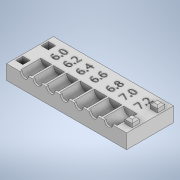
# Autodesk Inventor part: Measurement Test
Saved by Autodesk Inventor 2021 (Build 250183000, 183)
## iProperties
Created: 2021-06-07
Part Number: Measurement Test
Material: Generic
Document SubType Name: Modeling
Designer: Anton
Density: 1 g/cm^3
Appearance: Default
Author: Anton
Autodesk Inventor part; units mm, degrees
ref_plane "YZ Plane" through (0, 0, 0) normal (1, 0, 0) x (0, 1, 0)
ref_plane "XZ Plane" through (0, 0, 0) normal (0, 1, 0) x (-1, 0, 0)
ref_plane "XY Plane" through (0, 0, 0) normal (0, 0, 1) x (1, 0, 0)
sketch "Sketch1" plane through (0, 0, 0) normal (0, 1, 0) x (-1, 0, 0)
  line L0 (0, 0) -> (56, 0)
  line L1 (56, 0) -> (56, -15)
  line L2 (56, -15) -> (0, -15)
  line L3 (0, -15) -> (0, 0)
  dimension "d0" = 15
  dimension "d1" = 56
  constraints: 8 end point, 2 parallel, 1 horizontal, 1 perpendicular
  measures "d0" distance between parallel lines of L2 L0
  measures "d1" distance between parallel lines of L3 L1
extrude "Extrusion1" add sketch "Sketch1" along normal blind 8
sketch "Sketch2" plane through (-56, 0, 0) normal (0, 0, 1) x (1, 0, 0)
  line L0 (56, 8) -> (0, 8) projected
  circle A0 centre (4.85, 8) radius 3
  circle A1 centre (11.95, 8) radius 3.1
  circle A2 centre (19.25, 8) radius 3.2
  circle A3 centre (26.85, 8) radius 3.4
  circle A4 centre (34.75, 8) radius 3.5
  circle A5 centre (42.85, 8) radius 3.6
  line L1 (0, 0) -> (0, 8) projected
  line L2 (56, 0) -> (56, 8) projected
  circle A6 centre (51.15, 8) radius 3.7
  point P0 (47.45, 8)
  point P1 (54.85, 8)
  point P2 (39.25, 8)
  point P3 (46.45, 8)
  point P4 (31.25, 8)
  point P5 (38.25, 8)
  point P6 (23.45, 8)
  point P7 (30.25, 8)
  point P8 (16.05, 8)
  point P9 (22.45, 8)
  point P10 (8.85, 8)
  point P11 (15.05, 8)
  point P12 (1.85, 8)
  point P13 (7.85, 8)
  dimension "d4" = 6
  dimension "d5" = 6.2
  dimension "d6" = 6.4
  dimension "d7" = 6.8
  dimension "d8" = 7
  dimension "d9" = 7.2
  dimension "d10" = 4.85
  dimension "d12" = 1
  dimension "d13" = 1
  dimension "d14" = 1
  dimension "d15" = 1
  dimension "d17" = 1
  dimension "d18" = 7.4
  dimension "d19" = 1
  constraints: 7 centre point, 8 other
  measures "d4" diameter of A0
  measures "d5" diameter of A1
  measures "d6" diameter of A2
  measures "d7" diameter of A3
  measures "d8" diameter of A4
  measures "d9" diameter of A5
  measures "d10" distance from line of L1 A0.centre
  measures "d18" diameter of A6
extrude "Extrusion2" cut sketch "Sketch2" against normal blind 11 contours A6 L0 | A5 L0 | A4 L0 | A3 L0 | A2 L0 | A1 L0 | A0 L0 picked at (52.0195, 5.594) picked at (43.6691, 6.4548) picked at (34.8906, 6.8418) picked at (25.8719, 6.7218) picked at (18.6441, 7.1222) picked at (12.0746, 6.9742) picked at (5.7645, 7.296)
sketch "Sketch3" plane through (0, 8, 0) normal (0, 1, 0) x (1, 0, 0)
  line L0 (0, 0) -> (0, 15) projected
  line L1 (0, 15) -> (-55.9832, 15)
  line L2 (-55.9832, 15) -> (-55.9832, 24.7648)
  line L3 (-55.9832, 24.7648) -> (0, 24.7648)
  line L4 (0, 24.7648) -> (0, 15)
  constraints: 8 end point, 2 parallel, 1 horizontal, 1 perpendicular
extrude "Extrusion3" add sketch "Sketch3" against normal blind 8
sketch "Sketch5" plane through (0, 8, 0) normal (0, 1, 0) x (1, 0, 0)
  line L0 (-56, 15) -> (-56, 0) projected
  line L1 (-52.9832, 14) -> (-52.9832, 59.4153) construction
  line L2 (-52.9832, 59.4153) -> (-39.3814, 59.4153) construction
  line L3 (-39.3814, 59.4153) -> (-39.3814, 14) construction
  line L4 (-39.3814, 14) -> (-52.9832, 14) construction
  line L5 (-45.9832, 14) -> (-45.9832, 59.5193) construction
  line L6 (-45.9832, 59.5193) -> (-29.8115, 59.5193) construction
  line L7 (-29.8115, 59.5193) -> (-29.8115, 14) construction
  line L8 (-29.8115, 14) -> (-45.9832, 14) construction
  line L9 (-38.9832, 14) -> (-38.9832, 59.5309) construction
  line L10 (-38.9832, 59.5309) -> (-25.3814, 59.5309) construction
  line L11 (-25.3814, 59.5309) -> (-25.3814, 14) construction
  line L12 (-25.3814, 14) -> (-38.9832, 14) construction
  line L13 (-31.4832, 14) -> (-31.4832, 59.7081) construction
  line L14 (-31.4832, 59.7081) -> (-17.4293, 59.7081) construction
  line L15 (-17.4293, 59.7081) -> (-17.4293, 14) construction
  line L16 (-17.4293, 14) -> (-31.4832, 14) construction
  line L17 (-22.5355, 14) -> (-22.5355, 61.7081) construction
  line L18 (-22.5355, 61.7081) -> (-24.1276, 61.7081) construction
  line L19 (-24.1276, 61.7081) -> (-24.1276, 14) construction
  line L20 (-24.1276, 14) -> (-22.5355, 14) construction
  line L21 (-6.6524, 14) -> (-6.6524, 61.7081) construction
  line L22 (-6.6524, 61.7081) -> (6.9493, 61.7081) construction
  line L23 (6.9493, 61.7081) -> (6.9493, 14) construction
  line L24 (6.9493, 14) -> (-6.6524, 14) construction
  line L25 (-14.972, 14) -> (-14.972, 61.7081) construction
  line L26 (-14.972, 61.7081) -> (-1.3703, 61.7081) construction
  line L27 (-1.3703, 61.7081) -> (-1.3703, 14) construction
  line L28 (-1.3703, 14) -> (-14.972, 14) construction
  line L29 (-55.9832, 24.7648) -> (-55.9832, 15) projected
  line L30 (-48.15, 0) -> (-54.15, 0) projected
  line L31 (-40.95, 0) -> (-47.15, 0) projected
  line L32 (-33.55, 0) -> (-39.95, 0) projected
  line L33 (-25.75, 0) -> (-32.55, 0) projected
  line L34 (-9.55, 0) -> (-16.75, 0) projected
  line L35 (-1.15, 0) -> (-8.55, 0) projected
  line L36 (-17.75, 0) -> (-24.75, 0) projected
  line L37 (-5.9685, 16.8039) -> (-2.5681, 15.0729)
  line L38 (-2.5681, 15.0729) -> (-2.5681, 14.5024)
  line L39 (-2.5681, 14.5024) -> (-6.0981, 16.3306)
  line L40 (-6.0981, 16.3306) -> (-6.0981, 14.2658)
  line L41 (-6.0981, 14.2658) -> (-6.5681, 14.2658)
  line L42 (-6.5681, 14.2658) -> (-6.5681, 16.8039)
  line L43 (-6.5681, 16.8039) -> (-5.9685, 16.8039)
  line L44 (-2.5681, 18.1524) -> (-2.5681, 17.5105)
  line L45 (-2.5681, 17.5105) -> (-3.3331, 17.5105)
  line L46 (-3.3331, 17.5105) -> (-3.3331, 18.1524)
  line L47 (-3.3331, 18.1524) -> (-2.5681, 18.1524)
  line L48 (-2.5681, 21.4263) -> (-2.5681, 18.9595)
  line L49 (-2.5681, 18.9595) -> (-3.1354, 18.9595)
  spline S0 degree 2 poles (-3.1354, 18.9595) (-3.385, 19.2253) (-3.8485, 19.6985) (-4.0981, 19.9254) knots 0 0 0 1 2 2 2
  spline S1 degree 2 poles (-4.0981, 19.9254) (-4.6005, 20.3825) (-5.2035, 20.7164) (-5.5244, 20.7164) knots 0 0 0 1 2 2 2
  spline S2 degree 2 poles (-5.5244, 20.7164) (-5.6929, 20.7164) (-5.9458, 20.6126) (-6.0268, 20.5186) knots 0 0 0 1 2 2 2
  spline S3 degree 2 poles (-6.0268, 20.5186) (-6.1078, 20.4246) (-6.1889, 20.1783) (-6.1889, 20.0292) knots 0 0 0 1 2 2 2
  spline S4 degree 2 poles (-6.1889, 20.0292) (-6.1889, 19.8865) (-6.1176, 19.5948) (-6.0625, 19.4619) knots 0 0 0 1 2 2 2
  spline S5 degree 2 poles (-6.0625, 19.4619) (-6.0171, 19.3485) (-5.8874, 19.1378) (-5.842, 19.0729) knots 0 0 0 1 2 2 2
  line L50 (-5.842, 19.0729) -> (-5.842, 19.0438)
  line L51 (-5.842, 19.0438) -> (-6.4125, 19.0438)
  spline S6 degree 2 poles (-6.4125, 19.0438) (-6.4936, 19.2091) (-6.6524, 19.8023) (-6.6524, 20.0681) knots 0 0 0 1 2 2 2
  spline S7 degree 2 poles (-6.6524, 20.0681) (-6.6524, 20.6288) (-6.0592, 21.2609) (-5.5535, 21.2609) knots 0 0 0 1 2 2 2
  spline S8 degree 2 poles (-5.5535, 21.2609) (-5.3169, 21.2609) (-4.9214, 21.1507) (-4.7529, 21.0535) knots 0 0 0 1 2 2 2
  spline S9 degree 2 poles (-4.7529, 21.0535) (-4.5779, 20.9562) (-4.2343, 20.6742) (-4.0689, 20.5186) knots 0 0 0 1 2 2 2
  spline S10 degree 2 poles (-4.0689, 20.5186) (-3.7934, 20.2658) (-3.2035, 19.6467) (-3.0317, 19.4619) knots 0 0 0 1 2 2 2
  line L52 (-3.0317, 19.4619) -> (-3.0317, 21.4263)
  line L53 (-3.0317, 21.4263) -> (-2.5681, 21.4263)
  line L54 (-14.2913, 16.8039) -> (-10.891, 15.0729)
  line L55 (-10.891, 15.0729) -> (-10.891, 14.5024)
  line L56 (-10.891, 14.5024) -> (-14.421, 16.3306)
  line L57 (-14.421, 16.3306) -> (-14.421, 14.2658)
  line L58 (-14.421, 14.2658) -> (-14.891, 14.2658)
  line L59 (-14.891, 14.2658) -> (-14.891, 16.8039)
  line L60 (-14.891, 16.8039) -> (-14.2913, 16.8039)
  line L61 (-10.891, 18.1524) -> (-10.891, 17.5105)
  line L62 (-10.891, 17.5105) -> (-11.656, 17.5105)
  line L63 (-11.656, 17.5105) -> (-11.656, 18.1524)
  line L64 (-11.656, 18.1524) -> (-10.891, 18.1524)
  spline S11 degree 2 poles (-12.891, 21.4489) (-11.8148, 21.4489) (-10.8067, 20.8233) (-10.8067, 20.1718) knots 0 0 0 1 2 2 2
  spline S12 degree 2 poles (-10.8067, 20.1718) (-10.8067, 19.5105) (-11.8342, 18.8914) (-12.8877, 18.8914) knots 0 0 0 1 2 2 2
  spline S13 degree 2 poles (-12.8877, 18.8914) (-13.9704, 18.8914) (-14.972, 19.517) (-14.972, 20.1718) knots 0 0 0 1 2 2 2
  spline S14 degree 2 poles (-14.972, 20.1718) (-14.972, 20.8298) (-13.9347, 21.4489) (-12.891, 21.4489) knots 0 0 0 1 2 2 2
  spline S15 degree 2 poles (-11.6722, 20.7618) (-11.8699, 20.8395) (-12.4793, 20.9044) (-12.891, 20.9044) knots 0 0 0 1 2 2 2
  spline S16 degree 2 poles (-12.891, 20.9044) (-13.3026, 20.9044) (-13.9088, 20.8395) (-14.113, 20.7585) knots 0 0 0 1 2 2 2
  spline S17 degree 2 poles (-14.113, 20.7585) (-14.3172, 20.6775) (-14.5279, 20.3955) (-14.5279, 20.1718) knots 0 0 0 1 2 2 2
  spline S18 degree 2 poles (-14.5279, 20.1718) (-14.5279, 19.9481) (-14.3172, 19.6596) (-14.1065, 19.5754) knots 0 0 0 1 2 2 2
  spline S19 degree 2 poles (-14.1065, 19.5754) (-13.9023, 19.4943) (-13.2799, 19.436) (-12.8877, 19.436) knots 0 0 0 1 2 2 2
  spline S20 degree 2 poles (-12.8877, 19.436) (-12.4663, 19.436) (-11.9023, 19.4878) (-11.6819, 19.5721) knots 0 0 0 1 2 2 2
  spline S21 degree 2 poles (-11.6819, 19.5721) (-11.4744, 19.6499) (-11.2508, 19.9384) (-11.2508, 20.1718) knots 0 0 0 1 2 2 2
  spline S22 degree 2 poles (-11.2508, 20.1718) (-11.2508, 20.3922) (-11.4615, 20.6807) (-11.6722, 20.7618) knots 0 0 0 1 2 2 2
  spline S23 degree 2 poles (-19.7414, 16.8201) (-19.4334, 16.8201) (-18.9115, 16.6159) (-18.7365, 16.4441) knots 0 0 0 1 2 2 2
  spline S24 degree 2 poles (-18.7365, 16.4441) (-18.5517, 16.2658) (-18.3605, 15.8185) (-18.3605, 15.5494) knots 0 0 0 1 2 2 2
  spline S25 degree 2 poles (-18.3605, 15.5494) (-18.3605, 15.2804) (-18.542, 14.8363) (-18.7235, 14.6677) knots 0 0 0 1 2 2 2
  spline S26 degree 2 poles (-18.7235, 14.6677) (-18.9407, 14.4603) (-19.67, 14.2269) (-20.2017, 14.2269) knots 0 0 0 1 2 2 2
  spline S27 degree 2 poles (-20.2017, 14.2269) (-20.7235, 14.2269) (-21.5631, 14.4408) (-21.8743, 14.6645) knots 0 0 0 1 2 2 2
  spline S28 degree 2 poles (-21.8743, 14.6645) (-22.179, 14.8817) (-22.5193, 15.5689) (-22.5193, 16.0194) knots 0 0 0 1 2 2 2
  spline S29 degree 2 poles (-22.5193, 16.0194) (-22.5193, 16.1524) (-22.4934, 16.3857) (-22.4642, 16.4733) knots 0 0 0 1 2 2 2
  line L65 (-22.4642, 16.4733) -> (-21.9488, 16.4733)
  line L66 (-21.9488, 16.4733) -> (-21.9488, 16.4506)
  spline S30 degree 2 poles (-21.9488, 16.4506) (-21.9877, 16.376) (-22.0558, 16.1037) (-22.0558, 15.9481) knots 0 0 0 1 2 2 2
  spline S31 degree 2 poles (-22.0558, 15.9481) (-22.0558, 15.4489) (-21.3816, 14.8363) (-20.7203, 14.778) knots 0 0 0 1 2 2 2
  spline S32 degree 2 poles (-20.7203, 14.778) (-20.8532, 14.9692) (-20.9991, 15.3712) (-20.9991, 15.611) knots 0 0 0 1 2 2 2
  spline S33 degree 2 poles (-20.9991, 15.611) (-20.9991, 15.8444) (-20.9051, 16.1945) (-20.7624, 16.3857) knots 0 0 0 1 2 2 2
  spline S34 degree 2 poles (-20.7624, 16.3857) (-20.5971, 16.6062) (-20.085, 16.8201) (-19.7414, 16.8201) knots 0 0 0 1 2 2 2
  spline S35 degree 2 poles (-19.7187, 16.2755) (-19.965, 16.2755) (-20.2989, 16.1459) (-20.4156, 16.0032) knots 0 0 0 1 2 2 2
  spline S36 degree 2 poles (-20.4156, 16.0032) (-20.4999, 15.8963) (-20.555, 15.6305) (-20.555, 15.4911) knots 0 0 0 1 2 2 2
  spline S37 degree 2 poles (-20.555, 15.4911) (-20.555, 15.3031) (-20.4415, 14.9498) (-20.3346, 14.778) knots 0 0 0 1 2 2 2
  spline S38 degree 2 poles (-20.3346, 14.778) (-20.2762, 14.7747) (-20.166, 14.7682) (-20.0817, 14.7682) knots 0 0 0 1 2 2 2
  spline S39 degree 2 poles (-20.0817, 14.7682) (-19.6668, 14.7682) (-19.1579, 14.9303) (-19.025, 15.0535) knots 0 0 0 1 2 2 2
  spline S40 degree 2 poles (-19.025, 15.0535) (-18.8986, 15.1669) (-18.7981, 15.4133) (-18.7981, 15.5527) knots 0 0 0 1 2 2 2
  spline S41 degree 2 poles (-18.7981, 15.5527) (-18.7981, 15.8768) (-19.2584, 16.2755) (-19.7187, 16.2755) knots 0 0 0 1 2 2 2
  line L67 (-18.4448, 18.1524) -> (-18.4448, 17.5105)
  line L68 (-18.4448, 17.5105) -> (-19.2098, 17.5105)
  line L69 (-19.2098, 17.5105) -> (-19.2098, 18.1524)
  line L70 (-19.2098, 18.1524) -> (-18.4448, 18.1524)
  spline S42 degree 2 poles (-18.354, 20.1686) (-18.354, 19.8703) (-18.5323, 19.3809) (-18.6976, 19.2091) knots 0 0 0 1 2 2 2
  spline S43 degree 2 poles (-18.6976, 19.2091) (-18.8597, 19.0405) (-19.3005, 18.8655) (-19.5501, 18.8655) knots 0 0 0 1 2 2 2
  spline S44 degree 2 poles (-19.5501, 18.8655) (-19.8743, 18.8655) (-20.4188, 19.2123) (-20.5809, 19.5429) knots 0 0 0 1 2 2 2
  line L71 (-20.5809, 19.5429) -> (-20.5971, 19.5429)
  spline S45 degree 2 poles (-20.5971, 19.5429) (-20.7689, 19.248) (-21.1773, 18.9627) (-21.482, 18.9627) knots 0 0 0 1 2 2 2
  spline S46 degree 2 poles (-21.482, 18.9627) (-21.9326, 18.9627) (-22.5355, 19.6434) (-22.5355, 20.1686) knots 0 0 0 1 2 2 2
  spline S47 degree 2 poles (-22.5355, 20.1686) (-22.5355, 20.7131) (-21.965, 21.3712) (-21.5177, 21.3712) knots 0 0 0 1 2 2 2
  spline S48 degree 2 poles (-21.5177, 21.3712) (-21.2487, 21.3712) (-20.7235, 21.0567) (-20.5744, 20.7618) knots 0 0 0 1 2 2 2
  line L72 (-20.5744, 20.7618) -> (-20.5582, 20.7618)
  spline S49 degree 2 poles (-20.5582, 20.7618) (-20.3961, 21.1118) (-19.9294, 21.4716) (-19.5598, 21.4716) knots 0 0 0 1 2 2 2
  spline S50 degree 2 poles (-19.5598, 21.4716) (-19.0477, 21.4716) (-18.354, 20.7261) (-18.354, 20.1686) knots 0 0 0 1 2 2 2
  spline S51 degree 2 poles (-19.508, 20.9206) (-19.7543, 20.9206) (-20.0461, 20.7261) (-20.1952, 20.4506) knots 0 0 0 1 2 2 2
  spline S52 degree 2 poles (-20.1952, 20.4506) (-20.247, 20.3598) (-20.367, 20.0551) (-20.4448, 19.8639) knots 0 0 0 1 2 2 2
  spline S53 degree 2 poles (-20.4448, 19.8639) (-20.2989, 19.6434) (-19.8645, 19.4068) (-19.589, 19.4068) knots 0 0 0 1 2 2 2
  spline S54 degree 2 poles (-19.589, 19.4068) (-19.226, 19.4068) (-18.7527, 19.8444) (-18.7527, 20.175) knots 0 0 0 1 2 2 2
  spline S55 degree 2 poles (-18.7527, 20.175) (-18.7527, 20.5122) (-19.1579, 20.9206) (-19.508, 20.9206) knots 0 0 0 1 2 2 2
  spline S56 degree 2 poles (-21.5112, 20.846) (-21.7803, 20.846) (-22.1401, 20.4862) (-22.1401, 20.1653) knots 0 0 0 1 2 2 2
  spline S57 degree 2 poles (-22.1401, 20.1653) (-22.1401, 19.8736) (-21.8192, 19.5008) (-21.5436, 19.5008) knots 0 0 0 1 2 2 2
  spline S58 degree 2 poles (-21.5436, 19.5008) (-21.3459, 19.5008) (-21.0704, 19.6921) (-20.9602, 19.8833) knots 0 0 0 1 2 2 2
  spline S59 degree 2 poles (-20.9602, 19.8833) (-20.9148, 19.9643) (-20.7559, 20.3079) (-20.7106, 20.4473) knots 0 0 0 1 2 2 2
  spline S60 degree 2 poles (-20.7106, 20.4473) (-20.8888, 20.6807) (-21.2681, 20.846) (-21.5112, 20.846) knots 0 0 0 1 2 2 2
  spline S61 degree 2 poles (-28.7052, 16.8201) (-28.3973, 16.8201) (-27.8754, 16.6159) (-27.7003, 16.4441) knots 0 0 0 1 2 2 2
  spline S62 degree 2 poles (-27.7003, 16.4441) (-27.5156, 16.2658) (-27.3243, 15.8185) (-27.3243, 15.5494) knots 0 0 0 1 2 2 2
  spline S63 degree 2 poles (-27.3243, 15.5494) (-27.3243, 15.2804) (-27.5058, 14.8363) (-27.6874, 14.6677) knots 0 0 0 1 2 2 2
  spline S64 degree 2 poles (-27.6874, 14.6677) (-27.9046, 14.4603) (-28.6339, 14.2269) (-29.1655, 14.2269) knots 0 0 0 1 2 2 2
  spline S65 degree 2 poles (-29.1655, 14.2269) (-29.6874, 14.2269) (-30.5269, 14.4408) (-30.8381, 14.6645) knots 0 0 0 1 2 2 2
  spline S66 degree 2 poles (-30.8381, 14.6645) (-31.1428, 14.8817) (-31.4832, 15.5689) (-31.4832, 16.0194) knots 0 0 0 1 2 2 2
  spline S67 degree 2 poles (-31.4832, 16.0194) (-31.4832, 16.1524) (-31.4572, 16.3857) (-31.4281, 16.4733) knots 0 0 0 1 2 2 2
  line L73 (-31.4281, 16.4733) -> (-30.9127, 16.4733)
  line L74 (-30.9127, 16.4733) -> (-30.9127, 16.4506)
  spline S68 degree 2 poles (-30.9127, 16.4506) (-30.9516, 16.376) (-31.0196, 16.1037) (-31.0196, 15.9481) knots 0 0 0 1 2 2 2
  spline S69 degree 2 poles (-31.0196, 15.9481) (-31.0196, 15.4489) (-30.3454, 14.8363) (-29.6841, 14.778) knots 0 0 0 1 2 2 2
  spline S70 degree 2 poles (-29.6841, 14.778) (-29.817, 14.9692) (-29.9629, 15.3712) (-29.9629, 15.611) knots 0 0 0 1 2 2 2
  spline S71 degree 2 poles (-29.9629, 15.611) (-29.9629, 15.8444) (-29.8689, 16.1945) (-29.7263, 16.3857) knots 0 0 0 1 2 2 2
  spline S72 degree 2 poles (-29.7263, 16.3857) (-29.561, 16.6062) (-29.0488, 16.8201) (-28.7052, 16.8201) knots 0 0 0 1 2 2 2
  spline S73 degree 2 poles (-28.6825, 16.2755) (-28.9289, 16.2755) (-29.2627, 16.1459) (-29.3794, 16.0032) knots 0 0 0 1 2 2 2
  spline S74 degree 2 poles (-29.3794, 16.0032) (-29.4637, 15.8963) (-29.5188, 15.6305) (-29.5188, 15.4911) knots 0 0 0 1 2 2 2
  spline S75 degree 2 poles (-29.5188, 15.4911) (-29.5188, 15.3031) (-29.4054, 14.9498) (-29.2984, 14.778) knots 0 0 0 1 2 2 2
  spline S76 degree 2 poles (-29.2984, 14.778) (-29.24, 14.7747) (-29.1298, 14.7682) (-29.0456, 14.7682) knots 0 0 0 1 2 2 2
  spline S77 degree 2 poles (-29.0456, 14.7682) (-28.6306, 14.7682) (-28.1217, 14.9303) (-27.9888, 15.0535) knots 0 0 0 1 2 2 2
  spline S78 degree 2 poles (-27.9888, 15.0535) (-27.8624, 15.1669) (-27.7619, 15.4133) (-27.7619, 15.5527) knots 0 0 0 1 2 2 2
  spline S79 degree 2 poles (-27.7619, 15.5527) (-27.7619, 15.8768) (-28.2222, 16.2755) (-28.6825, 16.2755) knots 0 0 0 1 2 2 2
  line L75 (-27.4086, 18.1524) -> (-27.4086, 17.5105)
  line L76 (-27.4086, 17.5105) -> (-28.1736, 17.5105)
  line L77 (-28.1736, 17.5105) -> (-28.1736, 18.1524)
  line L78 (-28.1736, 18.1524) -> (-27.4086, 18.1524)
  spline S80 degree 2 poles (-28.7052, 21.4878) (-28.3973, 21.4878) (-27.8754, 21.2836) (-27.7003, 21.1118) knots 0 0 0 1 2 2 2
  spline S81 degree 2 poles (-27.7003, 21.1118) (-27.5156, 20.9335) (-27.3243, 20.4862) (-27.3243, 20.2172) knots 0 0 0 1 2 2 2
  spline S82 degree 2 poles (-27.3243, 20.2172) (-27.3243, 19.9481) (-27.5058, 19.5041) (-27.6874, 19.3355) knots 0 0 0 1 2 2 2
  spline S83 degree 2 poles (-27.6874, 19.3355) (-27.9046, 19.128) (-28.6339, 18.8947) (-29.1655, 18.8947) knots 0 0 0 1 2 2 2
  spline S84 degree 2 poles (-29.1655, 18.8947) (-29.6874, 18.8947) (-30.5269, 19.1086) (-30.8381, 19.3323) knots 0 0 0 1 2 2 2
  spline S85 degree 2 poles (-30.8381, 19.3323) (-31.1428, 19.5494) (-31.4832, 20.2366) (-31.4832, 20.6872) knots 0 0 0 1 2 2 2
  spline S86 degree 2 poles (-31.4832, 20.6872) (-31.4832, 20.8201) (-31.4572, 21.0535) (-31.4281, 21.141) knots 0 0 0 1 2 2 2
  line L79 (-31.4281, 21.141) -> (-30.9127, 21.141)
  line L80 (-30.9127, 21.141) -> (-30.9127, 21.1183)
  spline S87 degree 2 poles (-30.9127, 21.1183) (-30.9516, 21.0438) (-31.0196, 20.7715) (-31.0196, 20.6159) knots 0 0 0 1 2 2 2
  spline S88 degree 2 poles (-31.0196, 20.6159) (-31.0196, 20.1167) (-30.3454, 19.5041) (-29.6841, 19.4457) knots 0 0 0 1 2 2 2
  spline S89 degree 2 poles (-29.6841, 19.4457) (-29.817, 19.637) (-29.9629, 20.0389) (-29.9629, 20.2788) knots 0 0 0 1 2 2 2
  spline S90 degree 2 poles (-29.9629, 20.2788) (-29.9629, 20.5122) (-29.8689, 20.8622) (-29.7263, 21.0535) knots 0 0 0 1 2 2 2
  spline S91 degree 2 poles (-29.7263, 21.0535) (-29.561, 21.2739) (-29.0488, 21.4878) (-28.7052, 21.4878) knots 0 0 0 1 2 2 2
  spline S92 degree 2 poles (-28.6825, 20.9433) (-28.9289, 20.9433) (-29.2627, 20.8136) (-29.3794, 20.671) knots 0 0 0 1 2 2 2
  spline S93 degree 2 poles (-29.3794, 20.671) (-29.4637, 20.564) (-29.5188, 20.2982) (-29.5188, 20.1588) knots 0 0 0 1 2 2 2
  spline S94 degree 2 poles (-29.5188, 20.1588) (-29.5188, 19.9708) (-29.4054, 19.6175) (-29.2984, 19.4457) knots 0 0 0 1 2 2 2
  spline S95 degree 2 poles (-29.2984, 19.4457) (-29.24, 19.4425) (-29.1298, 19.436) (-29.0456, 19.436) knots 0 0 0 1 2 2 2
  spline S96 degree 2 poles (-29.0456, 19.436) (-28.6306, 19.436) (-28.1217, 19.5981) (-27.9888, 19.7212) knots 0 0 0 1 2 2 2
  spline S97 degree 2 poles (-27.9888, 19.7212) (-27.8624, 19.8347) (-27.7619, 20.081) (-27.7619, 20.2204) knots 0 0 0 1 2 2 2
  spline S98 degree 2 poles (-27.7619, 20.2204) (-27.7619, 20.5446) (-28.2222, 20.9433) (-28.6825, 20.9433) knots 0 0 0 1 2 2 2
  spline S99 degree 2 poles (-36.2052, 16.8201) (-35.8973, 16.8201) (-35.3754, 16.6159) (-35.2003, 16.4441) knots 0 0 0 1 2 2 2
  spline S100 degree 2 poles (-35.2003, 16.4441) (-35.0156, 16.2658) (-34.8243, 15.8185) (-34.8243, 15.5494) knots 0 0 0 1 2 2 2
  spline S101 degree 2 poles (-34.8243, 15.5494) (-34.8243, 15.2804) (-35.0058, 14.8363) (-35.1874, 14.6677) knots 0 0 0 1 2 2 2
  spline S102 degree 2 poles (-35.1874, 14.6677) (-35.4046, 14.4603) (-36.1339, 14.2269) (-36.6655, 14.2269) knots 0 0 0 1 2 2 2
  spline S103 degree 2 poles (-36.6655, 14.2269) (-37.1874, 14.2269) (-38.0269, 14.4408) (-38.3381, 14.6645) knots 0 0 0 1 2 2 2
  spline S104 degree 2 poles (-38.3381, 14.6645) (-38.6428, 14.8817) (-38.9832, 15.5689) (-38.9832, 16.0194) knots 0 0 0 1 2 2 2
  spline S105 degree 2 poles (-38.9832, 16.0194) (-38.9832, 16.1524) (-38.9572, 16.3857) (-38.9281, 16.4733) knots 0 0 0 1 2 2 2
  line L81 (-38.9281, 16.4733) -> (-38.4127, 16.4733)
  line L82 (-38.4127, 16.4733) -> (-38.4127, 16.4506)
  spline S106 degree 2 poles (-38.4127, 16.4506) (-38.4516, 16.376) (-38.5196, 16.1037) (-38.5196, 15.9481) knots 0 0 0 1 2 2 2
  spline S107 degree 2 poles (-38.5196, 15.9481) (-38.5196, 15.4489) (-37.8454, 14.8363) (-37.1841, 14.778) knots 0 0 0 1 2 2 2
  spline S108 degree 2 poles (-37.1841, 14.778) (-37.317, 14.9692) (-37.4629, 15.3712) (-37.4629, 15.611) knots 0 0 0 1 2 2 2
  spline S109 degree 2 poles (-37.4629, 15.611) (-37.4629, 15.8444) (-37.3689, 16.1945) (-37.2263, 16.3857) knots 0 0 0 1 2 2 2
  spline S110 degree 2 poles (-37.2263, 16.3857) (-37.061, 16.6062) (-36.5488, 16.8201) (-36.2052, 16.8201) knots 0 0 0 1 2 2 2
  spline S111 degree 2 poles (-36.1825, 16.2755) (-36.4289, 16.2755) (-36.7627, 16.1459) (-36.8794, 16.0032) knots 0 0 0 1 2 2 2
  spline S112 degree 2 poles (-36.8794, 16.0032) (-36.9637, 15.8963) (-37.0188, 15.6305) (-37.0188, 15.4911) knots 0 0 0 1 2 2 2
  spline S113 degree 2 poles (-37.0188, 15.4911) (-37.0188, 15.3031) (-36.9054, 14.9498) (-36.7984, 14.778) knots 0 0 0 1 2 2 2
  spline S114 degree 2 poles (-36.7984, 14.778) (-36.74, 14.7747) (-36.6298, 14.7682) (-36.5456, 14.7682) knots 0 0 0 1 2 2 2
  spline S115 degree 2 poles (-36.5456, 14.7682) (-36.1306, 14.7682) (-35.6217, 14.9303) (-35.4888, 15.0535) knots 0 0 0 1 2 2 2
  spline S116 degree 2 poles (-35.4888, 15.0535) (-35.3624, 15.1669) (-35.2619, 15.4133) (-35.2619, 15.5527) knots 0 0 0 1 2 2 2
  spline S117 degree 2 poles (-35.2619, 15.5527) (-35.2619, 15.8768) (-35.7222, 16.2755) (-36.1825, 16.2755) knots 0 0 0 1 2 2 2
  line L83 (-34.9086, 18.1524) -> (-34.9086, 17.5105)
  line L84 (-34.9086, 17.5105) -> (-35.6736, 17.5105)
  line L85 (-35.6736, 17.5105) -> (-35.6736, 18.1524)
  line L86 (-35.6736, 18.1524) -> (-34.9086, 18.1524)
  line L87 (-36.283, 21.5332) -> (-36.283, 21.0567)
  line L88 (-36.283, 21.0567) -> (-34.9086, 21.0567)
  line L89 (-34.9086, 21.0567) -> (-34.9086, 20.5413)
  line L90 (-34.9086, 20.5413) -> (-36.283, 20.5413)
  line L91 (-36.283, 20.5413) -> (-36.283, 18.7747)
  line L92 (-36.283, 18.7747) -> (-36.847, 18.7747)
  line L93 (-36.847, 18.7747) -> (-38.9086, 20.564)
  line L94 (-38.9086, 20.564) -> (-38.9086, 21.0567)
  line L95 (-38.9086, 21.0567) -> (-36.7141, 21.0567)
  line L96 (-36.7141, 21.0567) -> (-36.7141, 21.5332)
  line L97 (-36.7141, 21.5332) -> (-36.283, 21.5332)
  line L98 (-36.7141, 20.5413) -> (-38.2765, 20.5413)
  line L99 (-38.2765, 20.5413) -> (-36.7141, 19.1961)
  line L100 (-36.7141, 19.1961) -> (-36.7141, 20.5413)
  spline S118 degree 2 poles (-43.1955, 16.8201) (-42.8875, 16.8201) (-42.3657, 16.6159) (-42.1906, 16.4441) knots 0 0 0 1 2 2 2
  spline S119 degree 2 poles (-42.1906, 16.4441) (-42.0058, 16.2658) (-41.8146, 15.8185) (-41.8146, 15.5494) knots 0 0 0 1 2 2 2
  spline S120 degree 2 poles (-41.8146, 15.5494) (-41.8146, 15.2804) (-41.9961, 14.8363) (-42.1776, 14.6677) knots 0 0 0 1 2 2 2
  spline S121 degree 2 poles (-42.1776, 14.6677) (-42.3948, 14.4603) (-43.1242, 14.2269) (-43.6558, 14.2269) knots 0 0 0 1 2 2 2
  spline S122 degree 2 poles (-43.6558, 14.2269) (-44.1776, 14.2269) (-45.0172, 14.4408) (-45.3284, 14.6645) knots 0 0 0 1 2 2 2
  spline S123 degree 2 poles (-45.3284, 14.6645) (-45.6331, 14.8817) (-45.9734, 15.5689) (-45.9734, 16.0194) knots 0 0 0 1 2 2 2
  spline S124 degree 2 poles (-45.9734, 16.0194) (-45.9734, 16.1524) (-45.9475, 16.3857) (-45.9183, 16.4733) knots 0 0 0 1 2 2 2
  line L101 (-45.9183, 16.4733) -> (-45.4029, 16.4733)
  line L102 (-45.4029, 16.4733) -> (-45.4029, 16.4506)
  spline S125 degree 2 poles (-45.4029, 16.4506) (-45.4418, 16.376) (-45.5099, 16.1037) (-45.5099, 15.9481) knots 0 0 0 1 2 2 2
  spline S126 degree 2 poles (-45.5099, 15.9481) (-45.5099, 15.4489) (-44.8357, 14.8363) (-44.1744, 14.778) knots 0 0 0 1 2 2 2
  spline S127 degree 2 poles (-44.1744, 14.778) (-44.3073, 14.9692) (-44.4532, 15.3712) (-44.4532, 15.611) knots 0 0 0 1 2 2 2
  spline S128 degree 2 poles (-44.4532, 15.611) (-44.4532, 15.8444) (-44.3592, 16.1945) (-44.2165, 16.3857) knots 0 0 0 1 2 2 2
  spline S129 degree 2 poles (-44.2165, 16.3857) (-44.0512, 16.6062) (-43.5391, 16.8201) (-43.1955, 16.8201) knots 0 0 0 1 2 2 2
  spline S130 degree 2 poles (-43.1728, 16.2755) (-43.4191, 16.2755) (-43.753, 16.1459) (-43.8697, 16.0032) knots 0 0 0 1 2 2 2
  spline S131 degree 2 poles (-43.8697, 16.0032) (-43.954, 15.8963) (-44.0091, 15.6305) (-44.0091, 15.4911) knots 0 0 0 1 2 2 2
  spline S132 degree 2 poles (-44.0091, 15.4911) (-44.0091, 15.3031) (-43.8956, 14.9498) (-43.7887, 14.778) knots 0 0 0 1 2 2 2
  spline S133 degree 2 poles (-43.7887, 14.778) (-43.7303, 14.7747) (-43.6201, 14.7682) (-43.5358, 14.7682) knots 0 0 0 1 2 2 2
  spline S134 degree 2 poles (-43.5358, 14.7682) (-43.1209, 14.7682) (-42.612, 14.9303) (-42.4791, 15.0535) knots 0 0 0 1 2 2 2
  spline S135 degree 2 poles (-42.4791, 15.0535) (-42.3527, 15.1669) (-42.2522, 15.4133) (-42.2522, 15.5527) knots 0 0 0 1 2 2 2
  spline S136 degree 2 poles (-42.2522, 15.5527) (-42.2522, 15.8768) (-42.7125, 16.2755) (-43.1728, 16.2755) knots 0 0 0 1 2 2 2
  line L103 (-41.8989, 18.1524) -> (-41.8989, 17.5105)
  line L104 (-41.8989, 17.5105) -> (-42.6639, 17.5105)
  line L105 (-42.6639, 17.5105) -> (-42.6639, 18.1524)
  line L106 (-42.6639, 18.1524) -> (-41.8989, 18.1524)
  line L107 (-41.8989, 21.4263) -> (-41.8989, 18.9595)
  line L108 (-41.8989, 18.9595) -> (-42.4661, 18.9595)
  spline S137 degree 2 poles (-42.4661, 18.9595) (-42.7157, 19.2253) (-43.1793, 19.6985) (-43.4289, 19.9254) knots 0 0 0 1 2 2 2
  spline S138 degree 2 poles (-43.4289, 19.9254) (-43.9313, 20.3825) (-44.5342, 20.7164) (-44.8551, 20.7164) knots 0 0 0 1 2 2 2
  spline S139 degree 2 poles (-44.8551, 20.7164) (-45.0237, 20.7164) (-45.2765, 20.6126) (-45.3576, 20.5186) knots 0 0 0 1 2 2 2
  spline S140 degree 2 poles (-45.3576, 20.5186) (-45.4386, 20.4246) (-45.5196, 20.1783) (-45.5196, 20.0292) knots 0 0 0 1 2 2 2
  spline S141 degree 2 poles (-45.5196, 20.0292) (-45.5196, 19.8865) (-45.4483, 19.5948) (-45.3932, 19.4619) knots 0 0 0 1 2 2 2
  spline S142 degree 2 poles (-45.3932, 19.4619) (-45.3478, 19.3485) (-45.2182, 19.1378) (-45.1728, 19.0729) knots 0 0 0 1 2 2 2
  line L109 (-45.1728, 19.0729) -> (-45.1728, 19.0438)
  line L110 (-45.1728, 19.0438) -> (-45.7433, 19.0438)
  spline S143 degree 2 poles (-45.7433, 19.0438) (-45.8243, 19.2091) (-45.9832, 19.8023) (-45.9832, 20.0681) knots 0 0 0 1 2 2 2
  spline S144 degree 2 poles (-45.9832, 20.0681) (-45.9832, 20.6288) (-45.39, 21.2609) (-44.8843, 21.2609) knots 0 0 0 1 2 2 2
  spline S145 degree 2 poles (-44.8843, 21.2609) (-44.6477, 21.2609) (-44.2522, 21.1507) (-44.0836, 21.0535) knots 0 0 0 1 2 2 2
  spline S146 degree 2 poles (-44.0836, 21.0535) (-43.9086, 20.9562) (-43.565, 20.6742) (-43.3997, 20.5186) knots 0 0 0 1 2 2 2
  spline S147 degree 2 poles (-43.3997, 20.5186) (-43.1242, 20.2658) (-42.5342, 19.6467) (-42.3624, 19.4619) knots 0 0 0 1 2 2 2
  line L111 (-42.3624, 19.4619) -> (-42.3624, 21.4263)
  line L112 (-42.3624, 21.4263) -> (-41.8989, 21.4263)
  spline S148 degree 2 poles (-50.1987, 16.8201) (-49.8908, 16.8201) (-49.3689, 16.6159) (-49.1939, 16.4441) knots 0 0 0 1 2 2 2
  spline S149 degree 2 poles (-49.1939, 16.4441) (-49.0091, 16.2658) (-48.8178, 15.8185) (-48.8178, 15.5494) knots 0 0 0 1 2 2 2
  spline S150 degree 2 poles (-48.8178, 15.5494) (-48.8178, 15.2804) (-48.9994, 14.8363) (-49.1809, 14.6677) knots 0 0 0 1 2 2 2
  spline S151 degree 2 poles (-49.1809, 14.6677) (-49.3981, 14.4603) (-50.1274, 14.2269) (-50.659, 14.2269) knots 0 0 0 1 2 2 2
  spline S152 degree 2 poles (-50.659, 14.2269) (-51.1809, 14.2269) (-52.0204, 14.4408) (-52.3316, 14.6645) knots 0 0 0 1 2 2 2
  spline S153 degree 2 poles (-52.3316, 14.6645) (-52.6363, 14.8817) (-52.9767, 15.5689) (-52.9767, 16.0194) knots 0 0 0 1 2 2 2
  spline S154 degree 2 poles (-52.9767, 16.0194) (-52.9767, 16.1524) (-52.9507, 16.3857) (-52.9216, 16.4733) knots 0 0 0 1 2 2 2
  line L113 (-52.9216, 16.4733) -> (-52.4062, 16.4733)
  line L114 (-52.4062, 16.4733) -> (-52.4062, 16.4506)
  spline S155 degree 2 poles (-52.4062, 16.4506) (-52.4451, 16.376) (-52.5131, 16.1037) (-52.5131, 15.9481) knots 0 0 0 1 2 2 2
  spline S156 degree 2 poles (-52.5131, 15.9481) (-52.5131, 15.4489) (-51.8389, 14.8363) (-51.1776, 14.778) knots 0 0 0 1 2 2 2
  spline S157 degree 2 poles (-51.1776, 14.778) (-51.3105, 14.9692) (-51.4564, 15.3712) (-51.4564, 15.611) knots 0 0 0 1 2 2 2
  spline S158 degree 2 poles (-51.4564, 15.611) (-51.4564, 15.8444) (-51.3624, 16.1945) (-51.2198, 16.3857) knots 0 0 0 1 2 2 2
  spline S159 degree 2 poles (-51.2198, 16.3857) (-51.0545, 16.6062) (-50.5423, 16.8201) (-50.1987, 16.8201) knots 0 0 0 1 2 2 2
  spline S160 degree 2 poles (-50.176, 16.2755) (-50.4224, 16.2755) (-50.7563, 16.1459) (-50.8729, 16.0032) knots 0 0 0 1 2 2 2
  spline S161 degree 2 poles (-50.8729, 16.0032) (-50.9572, 15.8963) (-51.0123, 15.6305) (-51.0123, 15.4911) knots 0 0 0 1 2 2 2
  spline S162 degree 2 poles (-51.0123, 15.4911) (-51.0123, 15.3031) (-50.8989, 14.9498) (-50.7919, 14.778) knots 0 0 0 1 2 2 2
  spline S163 degree 2 poles (-50.7919, 14.778) (-50.7336, 14.7747) (-50.6234, 14.7682) (-50.5391, 14.7682) knots 0 0 0 1 2 2 2
  spline S164 degree 2 poles (-50.5391, 14.7682) (-50.1242, 14.7682) (-49.6152, 14.9303) (-49.4823, 15.0535) knots 0 0 0 1 2 2 2
  spline S165 degree 2 poles (-49.4823, 15.0535) (-49.3559, 15.1669) (-49.2554, 15.4133) (-49.2554, 15.5527) knots 0 0 0 1 2 2 2
  spline S166 degree 2 poles (-49.2554, 15.5527) (-49.2554, 15.8768) (-49.7157, 16.2755) (-50.176, 16.2755) knots 0 0 0 1 2 2 2
  line L115 (-48.9021, 18.1524) -> (-48.9021, 17.5105)
  line L116 (-48.9021, 17.5105) -> (-49.6671, 17.5105)
  line L117 (-49.6671, 17.5105) -> (-49.6671, 18.1524)
  line L118 (-49.6671, 18.1524) -> (-48.9021, 18.1524)
  spline S167 degree 2 poles (-50.9021, 21.4489) (-49.8259, 21.4489) (-48.8178, 20.8233) (-48.8178, 20.1718) knots 0 0 0 1 2 2 2
  spline S168 degree 2 poles (-48.8178, 20.1718) (-48.8178, 19.5105) (-49.8454, 18.8914) (-50.8989, 18.8914) knots 0 0 0 1 2 2 2
  spline S169 degree 2 poles (-50.8989, 18.8914) (-51.9815, 18.8914) (-52.9832, 19.517) (-52.9832, 20.1718) knots 0 0 0 1 2 2 2
  spline S170 degree 2 poles (-52.9832, 20.1718) (-52.9832, 20.8298) (-51.9459, 21.4489) (-50.9021, 21.4489) knots 0 0 0 1 2 2 2
  spline S171 degree 2 poles (-49.6833, 20.7618) (-49.8811, 20.8395) (-50.4905, 20.9044) (-50.9021, 20.9044) knots 0 0 0 1 2 2 2
  spline S172 degree 2 poles (-50.9021, 20.9044) (-51.3138, 20.9044) (-51.9199, 20.8395) (-52.1242, 20.7585) knots 0 0 0 1 2 2 2
  spline S173 degree 2 poles (-52.1242, 20.7585) (-52.3284, 20.6775) (-52.5391, 20.3955) (-52.5391, 20.1718) knots 0 0 0 1 2 2 2
  spline S174 degree 2 poles (-52.5391, 20.1718) (-52.5391, 19.9481) (-52.3284, 19.6596) (-52.1177, 19.5754) knots 0 0 0 1 2 2 2
  spline S175 degree 2 poles (-52.1177, 19.5754) (-51.9135, 19.4943) (-51.2911, 19.436) (-50.8989, 19.436) knots 0 0 0 1 2 2 2
  spline S176 degree 2 poles (-50.8989, 19.436) (-50.4775, 19.436) (-49.9135, 19.4878) (-49.693, 19.5721) knots 0 0 0 1 2 2 2
  spline S177 degree 2 poles (-49.693, 19.5721) (-49.4856, 19.6499) (-49.2619, 19.9384) (-49.2619, 20.1718) knots 0 0 0 1 2 2 2
  spline S178 degree 2 poles (-49.2619, 20.1718) (-49.2619, 20.3922) (-49.4726, 20.6807) (-49.6833, 20.7618) knots 0 0 0 1 2 2 2
  point P0 (0, 0)
  dimension "d25" = 3
  dimension "d26" = 10
  dimension "d27" = 14
  dimension "d28" = 14
  dimension "d29" = 17
  dimension "d30" = 14
  dimension "d31" = 14
  dimension "d32" = 24.5
  dimension "d34" = 14
  dimension "d35" = 14
  constraints: 14 other
  measures "d25" distance between parallel lines of L29 L1
  measures "d26" distance from line of L29.end L5
  measures "d27" distance between parallel lines of L30 L4
  measures "d28" distance between parallel lines of L31 L8
  measures "d29" distance between parallel lines of L29 L9
  measures "d30" distance between parallel lines of L32 L12
  measures "d31" distance between parallel lines of L33 L16
  measures "d32" distance between parallel lines of L29 L13
  measures "d34" distance between parallel lines of L35 L24
  measures "d35" distance between parallel lines of L36 L20
extrude "Extrusion4" cut sketch "Sketch5" against normal blind 0.5
sketch "Sketch6" plane through (-56, 0, 0) normal (0, 0, 1) x (1, 0, 0)
  line L0 (0, 0) -> (0, 8) projected
  line L1 (56, 0) -> (56, 8) projected
  line L2 (0, 8) -> (56, 8)
  line L3 (56, 8) -> (56, 0)
  line L4 (56, 0) -> (0, 0)
  line L5 (0, 0) -> (0, 8)
  constraints: 8 end point, 2 parallel, 1 horizontal, 1 perpendicular
extrude "Extrusion5" add sketch "Sketch6" along normal blind 1
sketch "Sketch7" plane through (-56, 0, -11) normal (0, 0, 1) x (1, 0, 0)
  line L0 (1.85, 8) -> (7.85, 8) projected
  circle A0 centre (4.85, 8) radius 2.25
  line L1 (8.85, 8) -> (15.05, 8) projected
  circle A1 centre (11.95, 8) radius 2.25
  line L2 (16.05, 8) -> (22.45, 8) projected
  circle A2 centre (19.25, 8) radius 2.25
  line L3 (23.45, 8) -> (30.25, 8) projected
  circle A3 centre (26.85, 8) radius 2.25
  line L4 (31.25, 8) -> (38.25, 8) projected
  circle A4 centre (34.75, 8) radius 2.25
  line L5 (39.25, 8) -> (46.45, 8) projected
  circle A5 centre (42.85, 8) radius 2.25
  line L6 (47.45, 8) -> (54.85, 8) projected
  circle A6 centre (51.15, 8) radius 2.25
  point P0 (56, 0)
  point P1 (53.4, 8)
  point P2 (48.9, 8)
  point P3 (45.1, 8)
  point P4 (40.6, 8)
  point P5 (37, 8)
  point P6 (32.5, 8)
  point P7 (29.1, 8)
  point P8 (24.6, 8)
  point P9 (21.5, 8)
  point P10 (17, 8)
  point P11 (14.2, 8)
  point P12 (9.7, 8)
  point P13 (7.1, 8)
  point P14 (2.6, 8)
  dimension "d40" = 4.5
  dimension "d41" = 4.5
  dimension "d42" = 4.5
  dimension "d43" = 4.5
  dimension "d44" = 4.5
  dimension "d45" = 4.5
  dimension "d46" = 4.5
  constraints: 7 centre point, 7 midpoint
  measures "d40" diameter of A0
  measures "d41" diameter of A1
  measures "d42" diameter of A2
  measures "d43" diameter of A3
  measures "d44" diameter of A4
  measures "d45" diameter of A5
  measures "d46" diameter of A6
extrude "Extrusion6" cut sketch "Sketch7" along normal blind 100 contours L0 A0 | L1 A1 | L2 A2 | L3 A3 | L4 A4 | L5 A5 | L6 A6 picked at (5.0263, 6.9069) picked at (12.6782, 6.586) picked at (19.1596, 7.2555) picked at (26.7596, 7.2555) picked at (34.6596, 7.2555) picked at (42.7596, 7.2555) picked at (51.0596, 7.2555)
sketch "Sketch8" plane through (0, 8, 0) normal (0, 1, 0) x (1, 0, 0)
  line L0 (-56, -1) -> (0, -1) projected
  line L1 (0, -1) -> (5, -1)
  line L2 (5, -1) -> (5, 24.7648)
  line L3 (5, 24.7648) -> (0, 24.7648)
  line L4 (0, 24.7648) -> (0, -1)
  line L5 (0, 24.7648) -> (-55.9832, 24.7648) projected
  line L6 (-55.9832, 24.7648) -> (-60.9832, 24.7648)
  line L7 (-60.9832, 24.7648) -> (-60.9832, -1)
  line L8 (-60.9832, -1) -> (-55.9832, -1)
  line L9 (-55.9832, -1) -> (-55.9832, 24.7648)
  point P0 (0, 0)
  dimension "d49" = 5
  dimension "d50" = 0
  dimension "d51" = 5
  constraints: 16 end point, 4 parallel, 2 horizontal, 2 perpendicular
  measures "d49" distance between parallel lines of L4 L2
  measures "d50" distance between parallel lines of L5 L3
  measures "d51" distance between parallel lines of L9 L7
extrude "Extrusion7" add sketch "Sketch8" against normal blind 8 contours L8 L7 L6 L9 L0 | L4 L3 L2 L1
sketch "Sketch9" plane through (0, 8, 0) normal (0, 1, 0) x (1, 0, 0)
  line L0 (-59.9832, 3) -> (-55.9832, 3)
  line L1 (-55.9832, 3) -> (-55.9832, 7)
  line L2 (-55.9832, 7) -> (-59.9832, 7)
  line L3 (-59.9832, 7) -> (-59.9832, 3)
  line L4 (-59.9832, 17) -> (-55.9832, 17)
  line L5 (-55.9832, 17) -> (-55.9832, 21)
  line L6 (-55.9832, 21) -> (-59.9832, 21)
  line L7 (-59.9832, 21) -> (-59.9832, 17)
  line L8 (0, 17) -> (4, 17)
  line L9 (4, 17) -> (4, 21)
  line L10 (4, 21) -> (0, 21)
  line L11 (0, 21) -> (0, 17)
  line L12 (0, 3) -> (4, 3)
  line L13 (4, 3) -> (4, 7)
  line L14 (4, 7) -> (0, 7)
  line L15 (0, 7) -> (0, 3)
  line L16 (-60.9832, 24.7648) -> (-60.9832, -1) projected
  line L17 (-53.4, -1) -> (-60.9832, -1) projected
  line L18 (5, -1) -> (5, 24.7648) projected
  point P0 (0, 0)
  dimension "d54" = 4
  dimension "d55" = 4
  dimension "d56" = 4
  dimension "d57" = 4
  dimension "d58" = 4
  dimension "d59" = 4
  dimension "d60" = 4
  dimension "d61" = 4
  dimension "d62" = 1
  dimension "d63" = 10
  dimension "d64" = 4
  dimension "d65" = 10
  dimension "d68" = 1
  dimension "d69" = 0
  constraints: 32 end point, 8 parallel, 4 horizontal, 4 perpendicular, 2 point on line
  measures "d54" distance between parallel lines of L1 L3
  measures "d55" distance between parallel lines of L0 L2
  measures "d56" distance between parallel lines of L7 L5
  measures "d57" distance between parallel lines of L4 L6
  measures "d58" distance between parallel lines of L9 L11
  measures "d59" distance between parallel lines of L8 L10
  measures "d60" distance between parallel lines of L12 L14
  measures "d61" distance between parallel lines of L13 L15
  measures "d62" distance between parallel lines of L16 L3
  measures "d63" distance between parallel lines of L2 L4
  measures "d64" distance between parallel lines of L17 L0
  measures "d65" distance between parallel lines of L8 L14
  measures "d68" distance between parallel lines of L18 L9
  measures "d69" distance between parallel lines of L9 L13
extrude "Extrusion8" add sketch "Sketch9" along normal blind 3 contours L11 L10 L9 L8 | L15 L14 L13 L12
sketch "Sketch10" plane through (0, 8, 0) normal (0, 1, 0) x (1, 0, 0)
  line L0 (-59.9832, 3) -> (-55.9832, 3)
  line L1 (-55.9832, 3) -> (-55.9832, 7)
  line L2 (-55.9832, 7) -> (-59.9832, 7)
  line L3 (-59.9832, 7) -> (-59.9832, 3)
  line L4 (-59.9832, 17) -> (-55.9832, 17)
  line L5 (-55.9832, 17) -> (-55.9832, 21)
  line L6 (-55.9832, 21) -> (-59.9832, 21)
  line L7 (-59.9832, 21) -> (-59.9832, 17)
  line L8 (-60.9832, 24.7648) -> (-60.9832, -1) projected
  line L9 (-53.4, -1) -> (-60.9832, -1) projected
  point P0 (0, 0)
  dimension "d72" = 1
  dimension "d73" = 1
  dimension "d74" = 4
  dimension "d75" = 4
  dimension "d76" = 4
  dimension "d77" = 4
  dimension "d78" = 4
  dimension "d79" = 10
  constraints: 16 end point, 4 parallel, 2 horizontal, 2 perpendicular
  measures "d72" distance between parallel lines of L8 L3
  measures "d73" distance between parallel lines of L8 L7
  measures "d74" distance between parallel lines of L4 L6
  measures "d75" distance between parallel lines of L7 L5
  measures "d76" distance between parallel lines of L0 L2
  measures "d77" distance between parallel lines of L1 L3
  measures "d78" distance between parallel lines of L9 L0
  measures "d79" distance between parallel lines of L4 L2
extrude "Extrusion9" cut sketch "Sketch10" against normal blind 5
chamfer "Chamfer1" distance 1 angle 45 8 edges at (4, 11, -19) (2, 11, -17) (2, 11, -21) (0, 11, -19) (0, 11, -5) (2, 11, -7) (2, 11, -3) (4, 11, -5)
body "Solid1"
